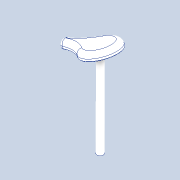
# Autodesk Inventor part: saddle
Saved by Autodesk Inventor 2021 (Build 250183000, 183)
## iProperties
Created: 2020-05-02
Part Number: saddle
Material: Aluminium 6082 T6
Document SubType Name: Modeling
Designer: Hannah
Appearance: Aluminum - Flat
Surface Area: 1171.49 cm^2
Volume: 730.873 cm^3
Vendor: Various
Description: saddle and seatpost
Size: [5]
Author: Hannah
Autodesk Inventor part; units mm, degrees
ref_plane "YZ Plane" through (0, 0, 0) normal (1, 0, 0) x (0, 1, 0)
ref_plane "XY Plane" through (0, 0, 0) normal (0, 0, 1) x (1, 0, 0)
sketch "Sketch1" plane through (0, 0, 0) normal (0, 1, 0) x (-1, 0, 0)
  circle A0 centre (0, 0) radius 13.5
  circle A1 centre (0, 0) radius 10.5
  dimension "d0" = 27
  dimension "d1" = 21
  constraints: 2 centre point, 2 coincident
  measures "d0" diameter of A0
  measures "d1" diameter of A1
extrude "Extrusion1" add sketch "Sketch1" against normal blind 400
ref_plane "Work Plane1" through (0, 0, 0) normal (-0.342, 0.9397, 0) x (0, 0, 1)
sketch "Sketch2" plane through (0, 0, 0) normal (-0.342, 0.9397, 0) x (-0.9397, -0.342, 0)
  ellipse E0 centre (0, 0) end of major axis (0, 13.5) minor radius 12.6859 projected
  arc A0 (45.088, 59.9339) -> (45.088, -59.9339) centre (0, 0) ccw
  arc A1 (155.9384, -19.978) -> (155.9384, 19.978) centre (155, 0) ccw
  arc A2 (155.9384, -19.978) -> (45.088, -59.9339) centre (165.3226, -219.7577) ccw
  line L0 (0, 0) -> (155, 0) construction
  arc A3 (45.088, 59.9339) -> (155.9384, 19.978) centre (165.3226, 219.7577) ccw
  point P0 (175, 0)
  point P1 (-75, 0)
  dimension "d7" = 150
  dimension "d8" = 40
  dimension "d9" = 155
  dimension "d10" = 200
  dimension "d15" = 250
  constraints: 10 point on circle, 4 centre point, 3 symmetric about line, 2 end point, 2 tangent, 1 coincident, 1 horizontal, 1 horizontal alignment, 2 other
  measures "d7" diameter of A0
  measures "d8" diameter of A1
  measures "d9" distance of point (0, 0) L0.end
  measures "d10" radius of A2
  measures "d15" distance of point (175, 0) point (-75, 0)
extrude "Extrusion2" add sketch "Sketch2" against normal mid plane 30 contours E0 | A3 A1 A2 A0
fillet "Fillet1" radius 20 4 edges at (65.3466, 39.7469, 0) (-96.754, -19.2529, -31.6072) (-169.5765, -45.7581, 0) (-96.754, -19.2529, 31.6072)
fillet "Fillet1" radius 2 4 edges at (-159.3159, -73.9489, 0) (-86.4934, -47.4437, -31.6072) (75.6072, 11.5561, 0) (-86.4934, -47.4437, 31.6072)
body "Solid1"
